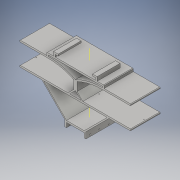
# Autodesk Inventor part: Test2
Saved by Autodesk Inventor 2016 (Build 200138000, 138)
## iProperties
Created: 2015-09-25
Part Number: Test2
Material: Generic
Document SubType Name: Modeling
Designer: fei
Density: 1 g/cm^3
Appearance: Default
Author: fei
Autodesk Inventor part; units mm, degrees
ref_plane "YZ Plane" through (0, 0, 0) normal (1, 0, 0) x (0, 1, 0)
ref_plane "XZ Plane" through (0, 0, 0) normal (0, 1, 0) x (-1, 0, 0)
ref_plane "XY Plane" through (0, 0, 0) normal (0, 0, 1) x (1, 0, 0)
sketch "Sketch1" plane through (0, 0, 0) normal (1, 0, 0) x (0, 1, 0)
  line L0 (38.1, 647.7) -> (-38.1, 647.7)
  line L1 (-38.1, 647.7) -> (-38.1, -647.7)
  line L2 (-38.1, -647.7) -> (38.1, -647.7)
  line L3 (38.1, -647.7) -> (38.1, 647.7)
  point P0 (0, 0)
  dimension "d0" = 1295.4
  dimension "d1" = 76.2
  dimension "d3" = 38.1
  dimension "d4" = 647.7
  constraints: 8 end point, 2 parallel, 1 horizontal, 1 perpendicular
  measures "d0" distance of L2.end L0.start
  measures "d1" distance of L0.start L0.end
  measures "d3" distance from line of point (0, 0) L1
  measures "d4" distance from line of L2 point (0, 0)
extrude "Extrusion1" add sketch "Sketch1" along normal blind 2463.8
sketch "Sketch2" plane through (0, 0, 0) normal (0, 0, 1) x (1, 0, 0)
  line L0 (0, -1130.3) -> (469.9, -1130.3)
  line L1 (469.9, -1130.3) -> (469.9, -1054.1)
  line L2 (469.9, -1054.1) -> (0, -1054.1)
  line L3 (0, -1054.1) -> (0, -1130.3)
  line L4 (0, -38.1) -> (2463.8, -38.1) projected
  line L5 (0, 0) -> (0, -1216.9003) construction
  dimension "d7" = 1092.2
  dimension "d8" = 76.2
  dimension "d9" = 469.9
  constraints: 10 end point, 2 parallel, 1 horizontal, 1 perpendicular, 1 point on line, 1 vertical
  measures "d7" distance between parallel lines of L0 L4
  measures "d8" distance of L0.end L1.end
  measures "d9" distance of L0.start L0.end
extrude "Extrusion2" add sketch "Sketch2" along normal mid plane 1295.4
sketch "Sketch4" plane through (0, -1054.1, 647.7) normal (0, 1, 0) x (1, 0, 0)
  line L0 (469.9, 1295.4) -> (469.9, 0) projected
  line L1 (469.9, 1295.4) -> (393.7, 1295.4)
  line L2 (393.7, 1295.4) -> (393.7, 0)
  line L3 (393.7, 0) -> (469.9, 0)
  line L4 (469.9, 0) -> (469.9, 1295.4)
  point P0 (0, 647.7)
  dimension "d12" = 76.2
  dimension "d13" = 1295.4
  constraints: 8 end point, 2 parallel, 1 horizontal, 1 perpendicular
  measures "d12" distance of L0.start L1.end
  measures "d13" distance of L1.end L2.end
sketch "Sketch6" plane through (0, 0, 0) normal (0, 0, 1) x (1, 0, 0)
  line L0 (469.9, -1054.1) -> (0, -1054.1) projected
  line L1 (0, -1054.1) -> (469.9, -1054.1) projected
  line L2 (431.8, -1054.1) -> (1447.8, -38.1)
  line L3 (0, -38.1) -> (2463.8, -38.1) projected
  line L4 (0, -1054.1) -> (1455.3911, -1054.1) construction
  line L5 (469.9, -1130.3) -> (469.9, -1054.1) construction
  point P0 (0, 0)
  dimension "d14" = 45
  dimension "d15" = 38.1
  constraints: 4 end point, 3 point on line
  measures "d14" angle of L4 L2
  measures "d15" distance from line of L5 L2.start
sweep "Sweep1" add profiles "Sketch4" path "Sketch6" path curves L2
sketch "Sketch7" plane through (0, -1130.3, 647.7) normal (0, -1, 0) x (1, 0, 0)
  line L0 (469.9, -1295.4) -> (469.9, 0) projected
  line L1 (393.7, -1295.4) -> (1409.7, -1295.4) projected
  line L2 (469.9, 0) -> (393.7, 0)
  line L3 (393.7, 0) -> (393.7, -1295.4)
  line L4 (393.7, -1295.4) -> (469.9, -1295.4)
  line L5 (469.9, -1295.4) -> (469.9, 0)
  point P0 (0, -647.7)
  constraints: 8 end point, 2 parallel, 1 horizontal, 1 perpendicular
extrude "Extrusion3" add sketch "Sketch7" along normal blind 203.2
sketch "Sketch8" plane through (0, 38.1, 647.7) normal (0, 1, 0) x (1, 0, 0)
  line L0 (0, 1295.4) -> (1409.7, 1295.4) projected
  line L1 (0, 0) -> (1409.7, 0) projected
  line L2 (254, 1295.4) -> (330.2, 1295.4)
  line L3 (330.2, 1295.4) -> (330.2, 0)
  line L4 (330.2, 0) -> (254, 0)
  line L5 (254, 0) -> (254, 1295.4)
  line L6 (0, 1295.4) -> (0, 0) projected
  point P0 (0, 647.7)
  dimension "d20" = 76.2
  dimension "d46" = 254
  constraints: 8 end point, 2 parallel, 2 point on line, 1 horizontal, 1 perpendicular
  measures "d20" distance of L2.start L2.end
  measures "d46" distance between parallel lines of L6 L5
sketch "Sketch9" plane through (0, 0, 0) normal (0, 0, 1) x (1, 0, 0)
  line L0 (0, 38.1) -> (2463.8, 38.1) projected
  line L1 (254, 38.1) -> (0, 292.1)
  point P0 (0, 0)
  dimension "d22" = 254
  dimension "d23" = 254
  constraints: 2 end point, 1 point on line
  measures "d22" distance from line of L0 L1.end
  measures "d23" horizontal distance of L1.start L1.end
sweep "Sweep2" add profiles "Sketch8" path "Sketch9" path curves L1 contours L0 L3 L1 L5
sketch "Sketch15" plane through (0, 292.1, 647.7) normal (0, 1, 0) x (1, 0, 0)
  line L0 (0, 0) -> (0, 1295.4) projected
  line L1 (76.2, 0) -> (76.2, 1295.4) projected
  line L2 (0, 1295.4) -> (76.2, 1295.4)
  line L3 (76.2, 1295.4) -> (76.2, 0)
  line L4 (76.2, 0) -> (0, 0)
  line L5 (0, 0) -> (0, 1295.4)
  point P0 (0, 647.7)
  constraints: 8 end point, 2 parallel, 1 horizontal, 1 perpendicular
extrude "Extrusion8" add sketch "Sketch15" along normal blind 381
sketch "Sketch16" plane through (0, 0, 0) normal (0, 0, 1) x (1, 0, 0)
  line L0 (2463.8, 38.1) -> (2463.8, -38.1) construction
  line L1 (2463.8, 0) -> (2463.8, 1154.2327) construction
  line L2 (2463.8, 927.1) -> (1193.8, 927.1)
  line L3 (330.2, 38.1) -> (2463.8, 38.1) projected
  line L4 (0, 673.1) -> (76.2, 673.1) projected
  arc A0 (1193.8, 927.1) -> (76.2, 673.1) centre (1193.8, -1658.62) ccw
  line L5 (2463.8, 927.1) -> (2463.8, 1003.3)
  line L6 (2463.8, 1003.3) -> (1193.8, 1003.3)
  line L7 (0, 673.1) -> (0, 711.2)
  arc A1 (1193.8, 1003.3) -> (0, 711.2) centre (1193.8, -1582.2543) ccw
  point P0 (0, 0)
  dimension "d49" = 1270
  dimension "d50" = 889
  dimension "d51" = 76.2
  dimension "d52" = 1270
  dimension "d53" = 38.1
  constraints: 10 end point, 4 point on circle, 2 centre point, 2 horizontal, 2 point on line, 2 tangent, 2 vertical, 1 midpoint
  measures "d49" distance of L2.start L2.end
  measures "d50" distance from line of L3 L2.start
  measures "d51" distance of L2.start L5.end
  measures "d52" distance of L5.end L6.end
  measures "d53" distance of L4.start L7.end
extrude "Extrusion9" add sketch "Sketch16" along normal mid plane 1295.4
mirror "Mirror4" about plane through (0, 0, 0) normal (1, 0, 0) of "Extrusion1", "Extrusion2", "Sweep1", "Extrusion3", "Sweep2", "Extrusion8", "Extrusion9"
sketch "Sketch17" plane through (1193.8, 1003.3, 647.7) normal (0, 1, 0) x (1, 0, 0)
  line L0 (-1117.6, 1295.4) -> (0, 1295.4) projected
  line L1 (1270, 0) -> (0, 0) projected
  line L2 (0, 1295.4) -> (76.2, 1295.4)
  line L3 (76.2, 1295.4) -> (76.2, 0)
  line L4 (76.2, 0) -> (0, 0)
  line L5 (0, 0) -> (0, 1295.4)
  point P0 (-1193.8, 647.7)
  point P1 (215.9, 0)
  dimension "d57" = 76.2
  constraints: 8 end point, 2 parallel, 1 horizontal, 1 perpendicular, 1 point on line
  measures "d57" distance of L0.end L2.end
extrude "Extrusion10" add sketch "Sketch17" along normal blind 127
sketch "Sketch18" plane through (1193.8, 1003.3, 647.7) normal (-1, 0, 0) x (0, 0, 1)
  line L0 (-1295.4, 0) -> (-1295.4, 127) projected
  line L1 (0, 0) -> (0, 127) projected
  line L2 (-1295.4, 127) -> (0, 127)
  line L3 (0, 127) -> (0, 50.8)
  line L4 (0, 50.8) -> (-1295.4, 50.8)
  line L5 (-1295.4, 50.8) -> (-1295.4, 127)
  point P0 (-647.7, -1003.3)
  dimension "d60" = 76.2
  constraints: 8 end point, 2 parallel, 1 horizontal, 1 perpendicular, 1 point on line
  measures "d60" distance of L1.end L3.end
extrude "Extrusion11" add sketch "Sketch18" along normal blind 1193.8
mirror "Mirror5" about plane through (0, 0, 0) normal (1, 0, 0) of "Extrusion10", "Extrusion11"
sketch "Sketch20" plane through (2463.8, 38.1, 647.7) normal (0, 1, 0) x (1, 0, 0)
  circle A0 centre (-2057.4, 647.7) radius 12.7
  circle A1 centre (-76.2, 647.7) radius 12.7
  line L0 (-2070.1, 1295.4) -> (-1054.1, 1295.4) projected
  line L1 (-2133.6, 0) -> (0, 0) projected
  line L2 (-2133.6, 1295.4) -> (-2133.6, 0) projected
  line L3 (0, 1295.4) -> (0, 0) projected
  point P0 (-2463.8, 647.7)
  dimension "d64" = 25.4
  dimension "d66" = 647.7
  dimension "d67" = 76.2
  dimension "d68" = 647.7
  dimension "d69" = 76.2
  dimension "d70" = 25.4
  constraints: 2 centre point
  measures "d64" diameter of A0
  measures "d66" distance from line of L1 A0.centre
  measures "d67" distance from line of L2 A0.centre
  measures "d68" distance from line of L1 A1.centre
  measures "d69" distance from line of L3 A1.centre
  measures "d70" diameter of A1
extrude "Extrusion12" cut sketch "Sketch20" against normal blind 76.2
mirror "Mirror6" about plane through (0, 0, 0) normal (1, 0, 0) of "Extrusion12"
fillet "Fillet1" radius 25.4 2 edges at (2463.8, 1003.3, 0) (2463.8, 927.1, 0)
fillet "Fillet2" radius 25.4 8 edges at (-2463.8, 1003.3, 0) (-2463.8, 927.1, 0) (1270, 1130.3, 0) (-1270, 1130.3, 0) (2463.8, 38.1, 0) (2463.8, -38.1, 0) (-2463.8, 38.1, 0) (-2463.8, -38.1, 0)
sketch "Sketch21" plane through (-469.9, -1333.5, -647.7) normal (-1, 0, 0) x (0, 0, 1)
  circle A0 centre (292.1, 76.2) radius 25.4
  line L0 (0, 279.4) -> (0, 0) projected
  line L1 (0, 0) -> (1295.4, 0) projected
  line L2 (292.1, 76.2) -> (860.7127, 76.2) construction
  circle A1 centre (698.5, 76.2) radius 25.4
  circle A2 centre (1104.9, 76.2) radius 25.4
  point P0 (647.7, 1333.5)
  dimension "d75" = 50.8
  dimension "d76" = 292.1
  dimension "d77" = 76.2
  dimension "d80" = 406.4
  constraints: 3 centre point, 2 end point, 2 horizontal, 4 other
  measures "d75" diameter of A0
  measures "d76" distance from line of L0 L2.start
  measures "d77" distance from line of L1 L2.start
  measures "d80" distance of L2.start A1.centre
extrude "Extrusion13" cut sketch "Sketch21" against normal through all
sketch "Sketch22" plane through (469.9, -1333.5, 647.7) normal (0, 0, 1) x (1, 0, 0)
  line L0 (-1295.4, 711.2) -> (355.6, 711.2) construction
  line L1 (-76.2, 279.4) -> (939.8, 1295.4) construction
  line L2 (-863.6, 279.4) -> (-1879.6, 1295.4) construction
  point P0 (-469.9, 1333.5)
  dimension "d87" = 1651
  constraints: 2 end point, 2 point on line, 1 horizontal
  measures "d87" distance of L0.start L0.end
sketch "Sketch23" plane through (393.7, -1054.1, -647.7) normal (-0.7071068, 0.7071068, 0) x (-0.7071068, -0.7071068, 0)
  line L0 (0, 1295.4) -> (-1436.841, 1295.4) construction
  line L1 (0, 0) -> (-1436.841, 0) construction
  line L2 (556.7759, 1295.4) -> (-610.6574, 1295.4) construction
  line L3 (-610.6574, 1295.4) -> (-610.6574, 0) construction
  line L4 (-839.2574, 393.7) -> (-610.6574, 393.7)
  line L5 (-610.6574, 393.7) -> (-610.6574, 647.7)
  line L6 (-610.6574, 647.7) -> (-839.2574, 647.7)
  line L7 (-839.2574, 647.7) -> (-839.2574, 393.7)
  point P0 (-466.9733, 647.7)
  dimension "d88" = 647.7
  dimension "d89" = 254
  dimension "d90" = 228.6
  constraints: 10 end point, 2 parallel, 2 perpendicular, 1 horizontal, 1 midpoint, 1 point on line
  measures "d88" distance from line of L1 L5.end
  measures "d89" distance of L6.end L4.start
  measures "d90" distance of L4.start L4.end
sketch "Sketch25" plane through (0, 0, 0) normal (0, 0, 1) x (1, 0, 0)
  line L0 (987.1446, -460.6554) -> (555.3446, -460.6554)
  point P0 (0, 0)
  dimension "d91" = 431.8
  constraints: 2 end point, 1 horizontal
  measures "d91" distance of L0.start L0.end
sweep "Sweep4" add profiles "Sketch23" path "Sketch25"
sketch "Sketch26" plane through (555.3446, -460.6554, 0) normal (0, 0, 1) x (1, 0, 0)
  line L0 (431.8, 0) -> (0, 0) projected
  line L1 (0, 0) -> (0, -161.6446)
  line L2 (270.1554, -161.6446) -> (-161.6446, -161.6446) projected
  line L3 (-161.6446, -161.6446) -> (0, 0) projected
  line L4 (-161.6446, -161.6446) -> (0, 0)
  point P0 (-555.3446, 460.6554)
  constraints: 4 end point, 1 collinear, 1 point on line, 1 vertical
extrude "Extrusion14" cut sketch "Sketch26" against normal blind 254
mirror "Mirror7" about plane through (0, 0, 0) normal (1, 0, 0) of "Sweep4", "Extrusion14"
sketch "Sketch28" plane through (1193.8, 1130.3, 647.7) normal (0, 1, 0) x (1, 0, 0)
  line L0 (-2603.5, 0) -> (215.9, 0) projected
  line L1 (-228.6, 0) -> (-228.6, 1016)
  line L2 (-206.6554, 901.7) -> (-638.4554, 901.7) projected
  line L3 (-228.6, 1016) -> (-304.8, 1016)
  line L4 (-304.8, 1016) -> (-304.8, 0)
  point P0 (-1193.8, 647.7)
  dimension "d106" = 76.2
  dimension "d107" = 1016
  dimension "d108" = 889
  constraints: 6 end point, 3 perpendicular, 2 point on line
  measures "d106" distance of L1.end L3.end
  measures "d107" distance of L1.start L1.end
  measures "d108" distance from line of point (-1193.8, 647.7) L4
extrude "Extrusion16" add sketch "Sketch28" along normal blind 177.8
sketch "Sketch31" plane through (889, 1130.3, -368.3) normal (-1, 0, 0) x (0, 0, 1)
  line L0 (0, 0) -> (0, 177.8) projected
  line L1 (1016, 0) -> (1016, 177.8) projected
  line L2 (0, 177.8) -> (1016, 177.8)
  line L3 (1016, 177.8) -> (1016, 101.6)
  line L4 (1016, 101.6) -> (0, 101.6)
  line L5 (0, 101.6) -> (0, 177.8)
  point P0 (368.3, -1130.3)
  dimension "d116" = 76.2
  constraints: 8 end point, 2 parallel, 1 horizontal, 1 perpendicular, 1 point on line
  measures "d116" distance of L1.end L3.end
extrude "Extrusion18" add sketch "Sketch31" along normal blind 127
mirror "Mirror8" about plane through (0, 0, 0) normal (1, 0, 0) of "Extrusion16", "Extrusion18"
body "Solid1"
